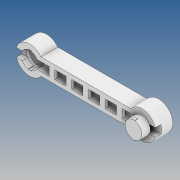
# Autodesk Inventor part: 2stopien
Saved by Autodesk Inventor 2022.3 (Build 263350000, 350)
## iProperties
Created: 2023-06-25
Part Number: 2stopien
Material: Tworzywo sztuczne ABS
Document SubType Name: Modeling
Designer: Chyba Ja
Density: 1.06 g/cm^3
Appearance: Gładki — biały
Author: Chyba Ja
Autodesk Inventor part; units mm, degrees
ref_plane "YZ Plane" through (0, 0, 0) normal (1, 0, 0) x (0, 1, 0)
ref_plane "XZ Plane" through (0, 0, 0) normal (0, 1, 0) x (-1, 0, 0)
ref_plane "XY Plane" through (0, 0, 0) normal (0, 0, 1) x (1, 0, 0)
sketch "Szkic1" plane through (0, 0, 0) normal (0, 0, 1) x (1, 0, 0)
  arc A0 (20, 15) -> (-20, 15) centre (0, 0) ccw
  line L0 (20, 15) -> (100, 15)
  line L1 (100, 15) -> (100, -15)
  line L2 (100, -15) -> (20, -15)
  arc A1 (180, -15) -> (180, 15) centre (200, 0) ccw
  line L3 (180, 15) -> (100, 15)
  line L4 (100, -15) -> (180, -15)
  arc A2 (-20, 15) -> (20, -15) centre (0, 0) ccw
  dimension "d0" = 50
  dimension "d1" = 30
  dimension "d2" = 200
  constraints: 10 end point, 6 point on circle, 5 symmetric about line, 4 coincident, 3 centre point, 1 horizontal, 1 parallel, 1 perpendicular, 1 point on line, 1 vertical alignment, 1 other
  measures "d0" diameter of A0
  measures "d1" distance between parallel lines of L2 L0
  measures "d2" distance of point (0, 0) point (200, 0)
extrude "kształt" add sketch "Szkic1" along normal blind 30
sketch "Szkic2" plane through (0, 0, 30) normal (0, 0, 1) x (1, 0, 0)
  arc A0 (20, 15) -> (20, -15) centre (0, 0) ccw projected
  line L0 (20, -15) -> (180, -15) projected
  arc A1 (180, -15) -> (180, 15) centre (200, 0) ccw projected
  line L1 (180, 15) -> (20, 15) projected
  line L2 (-23.8485, 7.5) -> (223.8485, 7.5)
  line L3 (223.8485, -7.5) -> (-73.8485, -7.5)
  point P0 (-23.8485, -7.5)
  dimension "d5" = 15
  constraints: 4 end point, 3 point on circle, 1 horizontal, 1 parallel, 1 vertical alignment
  measures "d5" distance between parallel lines of L3 L2
extrude "rowek na kable" cut sketch "Szkic2" against normal blind 10 contours L2 A1 L3 A0
sketch "Szkic3" plane through (0, 0, 30) normal (0, 0, 1) x (1, 0, 0)
  arc A0 (223.8485, 7.5) -> (180, 15) centre (200, 0) ccw projected
  circle A1 centre (200, 0) radius 15
  point P0 (0, 0)
  dimension "d8" = 30
  constraints: 1 centre point, 1 coincident
  measures "d8" diameter of A1
extrude "odstająćy cosik" add sketch "Szkic3" along normal blind 15
sketch "Szkic4" plane through (0, 0, 30) normal (0, 0, 1) x (1, 0, 0)
  circle A0 centre (0, 0) radius 15
  dimension "d11" = 30
  constraints: 1 centre point, 1 coincident
  measures "d11" diameter of A0
extrude "wgłebiający cosik" cut sketch "Szkic4" against normal blind 15
sketch "Szkic5" plane through (0, 0, 30) normal (0, 0, 1) x (1, 0, 0)
  arc A0 (12.9904, 7.5) -> (-12.9904, 7.5) centre (0, 0) ccw projected
  line L0 (12.9904, 7.5) -> (187.0096, 7.5) projected
  arc A1 (212.9904, 7.5) -> (187.0096, 7.5) centre (200, 0) ccw projected
  line L1 (212.9904, 7.5) -> (223.8485, 7.5) projected
  arc A2 (223.8485, 7.5) -> (180, 15) centre (200, 0) ccw projected
  line L2 (180, 15) -> (20, 15) projected
  arc A3 (20, 15) -> (-23.8485, 7.5) centre (0, 0) ccw projected
  line L3 (-23.8485, 7.5) -> (-12.9904, 7.5) projected
  arc A4 (-12.9904, -7.5) -> (12.9904, -7.5) centre (0, 0) ccw projected
  line L4 (-12.9904, -7.5) -> (-23.8485, -7.5) projected
  arc A5 (-23.8485, -7.5) -> (20, -15) centre (0, 0) ccw projected
  line L5 (20, -15) -> (180, -15) projected
  arc A6 (180, -15) -> (223.8485, -7.5) centre (200, 0) ccw projected
  line L6 (223.8485, -7.5) -> (212.9904, -7.5) projected
  arc A7 (187.0096, -7.5) -> (212.9904, -7.5) centre (200, 0) ccw projected
  line L7 (187.0096, -7.5) -> (12.9904, -7.5) projected
  line L8 (35, 7.5) -> (45, 7.5)
  line L9 (45, 7.5) -> (45, -7.5)
  line L10 (45, -7.5) -> (35, -7.5)
  line L11 (35, -7.5) -> (35, 7.5)
  arc A8 (-23.8485, -7.5) -> (20, -15) centre (0, 0) ccw projected
  line L12 (65, -7.5) -> (65, 7.5)
  line L13 (75, 7.5) -> (75, -7.5)
  line L14 (75, -7.5) -> (65, -7.5)
  line L15 (65, 7.5) -> (75, 7.5)
  line L16 (95, -7.5) -> (95, 7.5)
  line L17 (105, 7.5) -> (105, -7.5)
  line L18 (105, -7.5) -> (95, -7.5)
  line L19 (95, 7.5) -> (105, 7.5)
  line L20 (125, -7.5) -> (125, 7.5)
  line L21 (135, 7.5) -> (135, -7.5)
  line L22 (135, -7.5) -> (125, -7.5)
  line L23 (125, 7.5) -> (135, 7.5)
  line L24 (155, -7.5) -> (155, 7.5)
  line L25 (165, 7.5) -> (165, -7.5)
  line L26 (165, -7.5) -> (155, -7.5)
  line L27 (155, 7.5) -> (165, 7.5)
  arc A9 (223.8485, 7.5) -> (180, 15) centre (200, 0) ccw projected
  line L28 (0, 0) -> (100, 0) construction
  line L29 (100, -7.5) -> (100, 7.5) construction
  line L30 (100, 0) -> (200, 0) construction
  point P0 (35, -7.5)
  point P1 (75, -7.5)
  point P2 (75, 7.5)
  point P3 (65, 7.5)
  point P4 (165, -7.5)
  point P5 (165, 7.5)
  point P6 (155, 7.5)
  point P7 (155, -7.5)
  point P8 (135, -7.5)
  point P9 (135, 7.5)
  point P10 (125, 7.5)
  point P11 (105, -7.5)
  point P12 (105, 7.5)
  point P13 (95, 7.5)
  dimension "d15" = 10
  dimension "d18" = 30
  constraints: 46 end point, 4 horizontal, 3 midpoint, 2 parallel, 2 perpendicular, 2 point on line, 1 collinear, 33 other
  measures "d15" distance between parallel lines of L11 L9
  measures "d18" distance of L10.end L12.start
extrude "wzmocnienie" add sketch "Szkic5" against normal blind 5 contours L0 L9 L7 L11 | L0 L13 L7 L12 | L0 L17 L7 L16 | L0 L21 L7 L20 | L25 L7 L24 L0
sketch "Szkic6" plane through (200, 0, 45) normal (0, 0, 1) x (1, 0, 0)
  circle A0 centre (0, 0) radius 15 projected
  arc A1 (2.5, 15.8035) -> (2.5, -15.8035) centre (0, 0) ccw construction
  line L0 (-2.5, 15.8035) -> (2.5, 15.8035)
  line L1 (2.5, 15.8035) -> (2.5, 14.7902)
  line L2 (2.5, -15.8035) -> (-2.5, -15.8035)
  line L3 (-2.5, -15.8035) -> (-2.5, -14.7902)
  line L4 (2.5, 14.7902) -> (2.5, -14.7902) construction
  line L5 (-2.5, 14.7902) -> (-2.5, 15.8035)
  line L6 (-2.5, -14.7902) -> (-2.5, 14.7902) construction
  line L7 (2.5, -14.7902) -> (2.5, -15.8035)
  point P0 (-200, 0)
  dimension "d25" = 32
  dimension "d27" = 5
  constraints: 16 end point, 10 parallel, 8 point on circle, 3 perpendicular, 2 horizontal alignment, 1 centre point, 1 coincident, 1 horizontal
  measures "d25" diameter of A1
  measures "d27" distance between parallel lines of L6 L4
extrude "złobek" add sketch "Szkic6" against normal blind 5 contours A0 L5 L0 L1 | L7 L2 L3 A0
sketch "Szkic7" plane through (0, 0, 30) normal (0, 0, 1) x (1, 0, 0)
  circle A0 centre (0, 0) radius 16 construction
  line L0 (-2.5, 15.8035) -> (2.5, 15.8035)
  line L1 (2.5, -15.8035) -> (-2.5, -15.8035)
  arc A1 (12.9904, 7.5) -> (-12.9904, 7.5) centre (0, 0) ccw projected
  arc A2 (-12.9904, -7.5) -> (12.9904, -7.5) centre (0, 0) ccw projected
  line L2 (2.5, 15.8035) -> (2.5, 14.7902)
  line L3 (2.5, -14.7902) -> (2.5, -15.8035)
  line L4 (-2.5, -15.8035) -> (-2.5, -14.7902)
  line L5 (-2.5, 14.7902) -> (-2.5, 15.8035)
  arc A3 (2.5, 14.7902) -> (-2.5, 14.7902) centre (0, 0) ccw
  arc A4 (-2.5, -14.7902) -> (2.5, -14.7902) centre (0, 0) ccw
  point P0 (2.5, 15.2968)
  dimension "d30" = 32
  dimension "d32" = 5
  constraints: 12 end point, 11 point on circle, 5 parallel, 3 centre point, 2 coincident, 2 collinear, 2 perpendicular, 1 horizontal, 1 midpoint
  measures "d30" diameter of A0
  measures "d32" distance from line of L5 point (2.5, 15.297)
extrude "wklęsły żłobek" cut sketch "Szkic7" against normal up to surface (15 mm away)
sketch "Szkic8" plane through (0, 0, 15) normal (0, 0, 1) x (1, 0, 0)
  arc A0 (2.5, -14.7902) -> (2.5, 14.7902) centre (0, 0) ccw projected
  line L0 (2.5, 15.8035) -> (2.5, 14.7902) projected
  line L1 (-2.5, 15.8035) -> (2.5, 15.8035) projected
  line L2 (-2.5, 14.7902) -> (-2.5, 15.8035) projected
  arc A1 (-2.5, 14.7902) -> (-2.5, -14.7902) centre (0, 0) ccw projected
  line L3 (-2.5, -15.8035) -> (-2.5, -14.7902) projected
  line L4 (2.5, -15.8035) -> (-2.5, -15.8035) projected
  line L5 (2.5, -14.7902) -> (2.5, -15.8035) projected
  circle A2 centre (0, 0) radius 16
  circle A3 centre (0, 0) radius 15
  constraints: 2 centre point, 2 coincident, 2 point on circle, 1 concentric
extrude "rowek" cut sketch "Szkic8" along normal blind 5 contours A0 L0 A2 L5 | L3 A2 L2 A1
